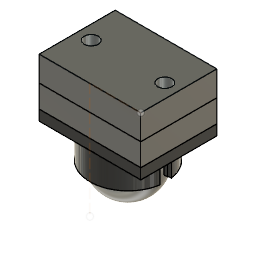
assembly (Autodesk Fusion 360 archive; units mm, degrees)
design "koło podporowe"
part number: 2025-11-20-20-36-54-064
part number: 2025-11-27-20-49-43-989
part number: 2025-11-27-20-56-08-265
Autodesk Fusion 360 part; units mm, degrees
note: some values were not read from the file. Set by a fixed rule: which face or edge a step refers to.
sketch "Szkic1" plane through (0, 0, 0) normal (0, 0, 1) x (1, 0, 0)
  line L0 (0, 0) -> (20.3, 0)
  line L1 (20.3, 0) -> (20.3, 15.2)
  line L2 (20.3, 15.2) -> (0, 15.2)
  line L3 (0, 15.2) -> (0, 0)
  dimension "d1" = 20.3
  dimension "d2" = 15.2
  constraint horizontal L0
  constraint vertical L1
  constraint horizontal L2
  constraint vertical L3
  constraint coincident L0.start L3.end
  measures "d1" distance of L0.start L0.end
  measures "d2" distance of L0.start L2.end
extrude "Wyciągnięcie proste1" add sketch "Szkic1" along normal blind 2.1 makes body 1
sketch "Szkic2" plane through (0, 0, 0) normal (0, 0, -1) x (1, 0, 0)
  line L0 (0, 0) -> (0, -15.2)
  line L1 (0, -15.2) -> (20.3, -15.2)
  line L2 (20.3, -15.2) -> (20.3, 0)
  line L3 (20.3, 0) -> (0, 0)
  circle A0 centre (2.8, -7.6) radius 1.15
  circle A1 centre (17.5, -7.6) radius 1.15
  dimension "d5" = 2.3
  dimension "d8" = 2.3
  measures "d5" diameter of A0
  measures "d8" diameter of A1
extrude "Wyciągnięcie proste2" cut sketch "Szkic2" against normal blind 4 contours A0 | A1 bodies 1
sketch "Szkic3" plane through (0, 0, 2.1) normal (0, 0, 1) x (-1, 0, 0)
  circle A0 centre (-2.8, -7.6) radius 1.15
  circle A1 centre (-17.5, -7.6) radius 1.15
  line L0 (0, -15.2) -> (0, 0)
  line L1 (0, 0) -> (-20.3, 0)
  line L2 (-20.3, 0) -> (-20.3, -15.2)
  line L3 (-20.3, -15.2) -> (0, -15.2)
  arc A2 (-17.6643, -8.7382) -> (-2.6357, -8.7382) centre (-10.15, -7.6) ccw
  arc A3 (-2.6357, -6.4618) -> (-17.6643, -6.4618) centre (-10.15, -7.6) ccw
  arc A4 (-3.9211, -6.6565) -> (-16.3789, -6.6565) centre (-10.15, -7.6) ccw
  arc A5 (-16.3789, -8.5435) -> (-3.9211, -8.5435) centre (-10.15, -7.6) ccw
  line L4 (-3.9211, -8.5435) -> (-3.294, -8.6385)
  line L5 (-3.9211, -6.6565) -> (-3.294, -6.5615)
  line L6 (-17.006, -6.5615) -> (-16.3789, -6.6565)
  line L7 (-17.006, -8.6385) -> (-16.3789, -8.5435)
  dimension "d13" = 15.2
  constraint coincident A1 A3.end
  constraint coincident A1 A2.start
  constraint coincident A0 A2.end
  constraint coincident A0 A3.start
  constraint concentric A2 A3
  constraint parallel L4 L6
  constraint parallel L5 L7
  constraint coincident A0 L4.end
  constraint coincident A0 L5.end
  constraint coincident A1 L7.start
  constraint coincident A1 L6.start
  measures "d13" diameter of A2
extrude "Wyciągnięcie proste3" add sketch "Szkic3" along normal blind 5.4 contours A0 A1 A3 A4 L5 L6 | A0 A1 A2 A5 L4 L7 bodies 1
sketch "Szkic4" plane through (0, 0, 0) normal (0, 0, -1) x (1, 0, 0)
  circle A0 centre (2.8, -7.6) radius 1.15
  circle A1 centre (17.5, -7.6) radius 1.15
  line L0 (0, 0) -> (0, -15.2)
  line L1 (0, -15.2) -> (20.3, -15.2)
  line L2 (20.3, -15.2) -> (20.3, 0)
  line L3 (20.3, 0) -> (0, 0)
  circle A2 centre (10.15, -7.6) radius 3.8
  dimension "d20" = 7.6
  measures "d20" diameter of A2
extrude "Wyciągnięcie proste4" cut sketch "Szkic4" against normal blind 4 contours A2 bodies 1
sphere "Prymityw sfery1" cut diameter 12.7 placed x (1, 0, 0) y (0, -1, 0) z (0, 0, -1) at (10.15, 7.6, 0) bodies 1
sphere "Prymityw sfery2" add diameter 12.7 placed x (1, 0, 0) y (0, -1, 0) z (0, 0, -1) at (10.15, 7.0726, 0) separate body makes body 2
move_body "Przesuń powierzchnię1" bodies 2 to x (1, 0, 0) y (0, 1, 0) z (0, 0, 1) at (0, 0, 7.15) on bodies 2
move_body "Przesuń powierzchnię2" bodies 2 to x (1, 0, 0) y (0, 1, 0) z (0, 0, 1) at (0, 0.5, 0) on bodies 2
sketch "Szkic7" plane through (0, 0, 0) normal (0, 1, 0) x (1, 0, 0)
sketch "Szkic8" plane through (0, 0, 0) normal (0, 0, 1) x (1, 0, 0)
  line L0 (0, 0) -> (20.3, 0)
  line L1 (20.3, 0) -> (20.3, 15.2)
  line L2 (20.3, 15.2) -> (0, 15.2)
  line L3 (0, 15.2) -> (0, 0)
  circle A0 centre (2.8, 7.6) radius 1.15
  arc A1 (3.8219, 8.1274) -> (3.8219, 7.0726) centre (2.8, 7.6) ccw
  circle A2 centre (17.5, 7.6) radius 1.15
  arc A3 (16.4781, 7.0726) -> (16.4781, 8.1274) centre (17.5, 7.6) ccw
  dimension "d27" = 20.3
  dimension "d28" = 15.2
  constraint horizontal L0
  constraint vertical L1
  constraint horizontal L2
  constraint vertical L3
  constraint coincident L0.start L3.end
  constraint tangent A0 A1
  constraint tangent A2 A3
  measures "d27" distance of L0.start L0.end
  measures "d28" distance of L0.start L2.end
ref_plane "Płaszczyzna konstrukcyjna1" through (10.15, 7.6, -1.5) normal (0, 0, -1) x (-1, 0, 0)
sketch "Szkic9" plane through (0, 0, -1.5) normal (0, 0, -1) x (-1, 0, 0)
  line L0 (0, 0) -> (-20.3, 0)
  line L1 (-20.3, 0) -> (-20.3, 15.2)
  line L2 (-20.3, 15.2) -> (0, 15.2)
  line L3 (0, 15.2) -> (0, 0)
  dimension "d32" = 20.3
  dimension "d33" = 15.2
  constraint horizontal L0
  constraint vertical L1
  constraint horizontal L2
  constraint vertical L3
  constraint coincident L0.start L3.end
  measures "d32" distance of L0.start L0.end
  measures "d33" distance of L0.start L2.end
extrude "Wyciągnięcie proste1'" add sketch "Szkic8" against normal blind 4.5 separate body makes body 3 in component "Component'"
ref_plane "Płaszczyzna konstrukcyjna2" through (10.15, 7.6, -4.5) normal (0, 0, -1) x (-1, 0, 0)
sketch "Szkic10" plane through (0, 0, -4.5) normal (0, 0, -1) x (-1, 0, 0)
  circle A0 centre (-2.8, 7.6) radius 1.4
  circle A1 centre (-17.5, 7.6) radius 1.4
  circle A2 centre (-17.5, 7.6) radius 1.15
  line L0 (-20.3, 0) -> (0, 0)
  line L1 (0, 0) -> (0, 15.2)
  line L2 (0, 15.2) -> (-20.3, 15.2)
  line L3 (-20.3, 15.2) -> (-20.3, 0)
  dimension "d39" = 2.8
  dimension "d40" = 2.8
  dimension "d41" = 20.3
  dimension "d42" = 15.2
  constraint concentric A1 A2
  constraint horizontal L0
  constraint vertical L1
  constraint horizontal L2
  constraint vertical L3
  measures "d39" diameter of A0
  measures "d40" diameter of A1
  measures "d41" distance of L0.start L0.end
  measures "d42" distance of L0.start L2.end
extrude "Wyciągnięcie proste1''" add sketch "Szkic10" along normal blind 5 separate body contours L0 L1 L2 L3 makes body 4 in component "do_druku"
move_body "Przesuń1" bodies 1 2 to x (-1, 0, 0) y (0, 1, 0) z (0, 0, -1) at (20.3, 0, 14.2)
move_body "Przesuń1'" bodies 4 to x (-1, 0, 0) y (0, 1, 0) z (0, 0, -1) at (20.3, 0, 14.2) in component "do_druku"
move_body "Przesuń1''" bodies 3 to x (-1, 0, 0) y (0, 1, 0) z (0, 0, -1) at (20.3, 0, 14.2) in component "Component'"
sketch "Szkic11" plane through (0, 0, 0) normal (0, 1, 0) x (1, 0, 0)
  line L0 (20.3, -23.7) -> (10.15, -23.7) construction
  line L1 (10.15, -23.7) -> (10.15, -0.7) construction
  dimension "d45" = 10.15
  dimension "d46" = 23
  constraint horizontal L0
  constraint vertical L1
  measures "d45" distance of L0.start L0.end
  measures "d46" distance of L0.end L1.end
sketch "Szkic12" plane through (0, 0, 23.7) normal (0, 0, 1) x (-1, 0, 0)
  circle A0 centre (-2.8, -7.6) radius 1.4
  circle A1 centre (-17.5, -7.6) radius 1.4
  line L0 (0, -15.2) -> (0, 0)
  line L1 (0, 0) -> (-20.3, 0)
  line L2 (-20.3, 0) -> (-20.3, -15.2)
  line L3 (-20.3, -15.2) -> (0, -15.2)
sketch "Szkic13" plane through (0, 0, 0) normal (0, 1, 0) x (1, 0, 0)
component "Component'" placed x (1, 0, 0) y (0, 1, 0) z (0, 0, 1) at (0, 0, 0)
component "do_druku" placed x (1, 0, 0) y (0, 1, 0) z (0, 0, 1) at (0, 0, 0)
named bodies: "kolo podporowe"

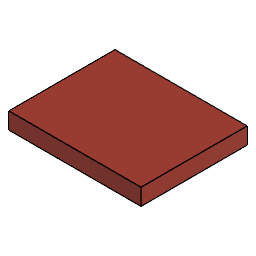
design "stepdown_5V"
part number: 2025-11-21-11-59-02-291
part number: 2025-11-29-20-27-12-206
Autodesk Fusion 360 part; units mm, degrees
sketch "Szkic1" plane through (0, 0, 0) normal (0, 0, 1) x (1, 0, 0)
  line L0 (0, 0) -> (12.7, 0)
  line L1 (12.7, 0) -> (12.7, 10.2)
  line L2 (12.7, 10.2) -> (0, 10.2)
  line L3 (0, 10.2) -> (0, 0)
  dimension "d1" = 12.7
  dimension "d2" = 10.2
  constraint horizontal L0
  constraint vertical L1
  constraint horizontal L2
  constraint vertical L3
  constraint coincident L0.start L3.end
  measures "d1" distance of L0.start L0.end
  measures "d2" distance of L0.start L2.end
extrude "Wyciągnięcie proste1" add sketch "Szkic1" along normal blind 1.6 makes body 1
copy_body "Bryła->Komponent1" bodies 1 removing the originals makes body 2 in component "Component"
component "Component" placed x (1, 0, 0) y (0, 1, 0) z (0, 0, 1) at (0, 0, 0)

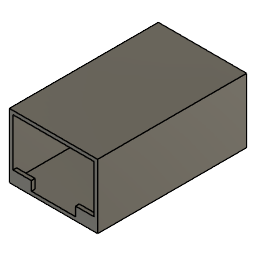
design "koszyk na koszyk"
part number: 2025-11-27-19-42-51-452
part number: 2025-11-29-21-01-25-605
Autodesk Fusion 360 part; units mm, degrees
sketch "Szkic1" plane through (0, 0, 0) normal (0, 0, 1) x (1, 0, 0)
  line L0 (0, 0) -> (48, 0)
  line L1 (48, 0) -> (48, 81)
  line L2 (48, 81) -> (0, 81)
  line L3 (0, 81) -> (0, 0)
  dimension "d1" = 48
  dimension "d2" = 81
  constraint horizontal L0
  constraint vertical L1
  constraint horizontal L2
  constraint vertical L3
  constraint coincident L0.start L3.end
  measures "d1" distance of L0.start L0.end
  measures "d2" distance of L0.start L2.end
extrude "Wyciągnięcie proste1" add sketch "Szkic1" along normal blind 2 makes body 1
ref_plane "Płaszczyzna konstrukcyjna1" through (0, 0, 2) normal (0, 0, 1) x (1, 0, 0)
sketch "Szkic2" plane through (0, 0, 2) normal (0, 0, 1) x (1, 0, 0)
  line L0 (0, 2) -> (2, 2) construction
  line L1 (0, 0) -> (48, 0)
  line L2 (48, 0) -> (48, 81)
  line L3 (48, 81) -> (0, 81)
  line L4 (0, 81) -> (0, 0)
  line L5 (2, 2) -> (12, 2)
  line L6 (12, 2) -> (12, 0)
  line L7 (12, 0) -> (2, 0)
  line L8 (2, 0) -> (2, 2)
  line L9 (46, 2) -> (36, 2)
  line L10 (36, 2) -> (36, 0)
  line L11 (36, 0) -> (46, 0)
  line L12 (46, 0) -> (46, 2)
  line L13 (0, 0) -> (2, 0)
  line L14 (2, 0) -> (2, 81)
  line L15 (2, 81) -> (0, 81)
  line L16 (0, 81) -> (0, 0)
  line L17 (48, 0) -> (46, 0)
  line L18 (46, 0) -> (46, 81)
  line L19 (46, 81) -> (48, 81)
  line L20 (48, 81) -> (48, 0)
  dimension "d8" = 44
  dimension "d10" = 48
  dimension "d11" = 81
  dimension "d12" = 10
  dimension "d13" = 2
  dimension "d16" = 10
  dimension "d19" = 81
  dimension "d22" = 81
  constraint horizontal L1
  constraint vertical L2
  constraint horizontal L3
  constraint vertical L4
  constraint coincident L1.start L4.end
  constraint horizontal L5
  constraint vertical L6
  constraint horizontal L7
  constraint vertical L8
  constraint horizontal L9
  constraint vertical L10
  constraint horizontal L11
  constraint vertical L12
  constraint horizontal L13
  constraint vertical L14
  constraint horizontal L15
  constraint vertical L16
  constraint horizontal L17
  constraint vertical L18
  constraint horizontal L19
  constraint vertical L20
  measures "d8" distance of L0.end L9.start
  measures "d10" distance of L1.start L1.end
  measures "d11" distance of L1.start L3.end
  measures "d12" distance of L0.end L5.end
  measures "d13" distance of L0.end L7.end
  measures "d16" distance of L9.start L9.end
  measures "d19" distance of L1.start L3.end
  measures "d22" distance of L1.end L2.end
extrude "Wyciągnięcie proste2" add sketch "Szkic2" along normal blind 5 contours L1 L5 L6 L7 L8 L14 bodies 1
extrude "Wyciągnięcie proste3" add sketch "Szkic2" along normal blind 5 contours L1 L9 L10 L11 L12 L18 bodies 1
extrude "Wyciągnięcie proste4" add sketch "Szkic2" along normal blind 31 contours L1 L3 L4 L8 L13 L14 L15 L16 bodies 1
extrude "Wyciągnięcie proste5" add sketch "Szkic2" along normal blind 31 contours L1 L2 L3 L12 L17 L18 L19 L20 bodies 1
ref_plane "Płaszczyzna konstrukcyjna2" through (0, 0, 33) normal (0, 0, 1) x (1, 0, 0)
sketch "Szkic3" plane through (0, 0, 33) normal (0, 0, 1) x (1, 0, 0)
  line L0 (0, 0) -> (48, 0)
  line L1 (48, 0) -> (48, 81)
  line L2 (48, 81) -> (0, 81)
  line L3 (0, 81) -> (0, 0)
  dimension "d26" = 48
  dimension "d27" = 81
  constraint horizontal L0
  constraint vertical L1
  constraint horizontal L2
  constraint vertical L3
  constraint coincident L0.start L3.end
  measures "d26" distance of L0.start L0.end
  measures "d27" distance of L0.start L2.end
extrude "Wyciągnięcie proste6" add sketch "Szkic3" along normal blind 2 bodies 1
copy_body "Bryła->Komponent1" bodies 1 removing the originals makes body 2 in component "Component"
component "Component" placed x (1, 0, 0) y (0, 1, 0) z (0, 0, 1) at (0, 0, 0)

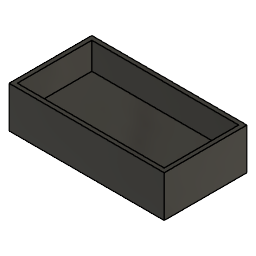
design "koszyk na baterie"
part number: 2025-11-20-20-18-58-786
part number: 2025-11-29-21-09-07-415
Autodesk Fusion 360 part; units mm, degrees
sketch "Szkic1" plane through (0, 0, 0) normal (0, 0, 1) x (1, 0, 0)
  line L0 (0, 0) -> (75, 0)
  line L1 (75, 0) -> (75, 40)
  line L2 (75, 40) -> (0, 40)
  line L3 (0, 40) -> (0, 0)
  dimension "d1" = 75
  dimension "d2" = 40
  constraint horizontal L0
  constraint vertical L1
  constraint horizontal L2
  constraint vertical L3
  constraint coincident L0.start L3.end
  measures "d1" distance of L0.start L0.end
  measures "d2" distance of L0.start L2.end
extrude "Wyciągnięcie proste1" add sketch "Szkic1" along normal blind 20 makes body 1
shell "Skorupa1" thickness 2 removed faces 1 at (25, 26.6667, 20) on bodies 1
extrude "Wyciągnięcie proste2" add 1 faces at (25.6667, 14, 2) along direction (0, 0, 1) blind 5 on bodies 1 bodies 1
copy_body "Bryła->Komponent1" bodies 1 removing the originals makes body 2 in component "koszyk"
component "koszyk" placed x (1, 0, 0) y (0, 1, 0) z (0, 0, 1) at (0, 0, 0)
named bodies: "koszyk"

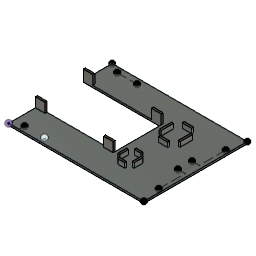
design "Podstawa"
part number: 2025-11-28-16-54-35-976
part number: 2025-11-29-20-28-41-836
Autodesk Fusion 360 part; units mm, degrees
other "Kontekst pochodny1"
sketch "Szkic1" plane through (0, 0, 0) normal (0, 0, 1) x (1, 0, 0)
  line L0 (0, 0) -> (141, 0)
  line L1 (141, 0) -> (141, 108)
  line L2 (141, 108) -> (0, 108)
  line L3 (0, 108) -> (0, 78)
  line L4 (0, 78) -> (81, 78)
  line L5 (81, 78) -> (81, 30)
  line L6 (81, 30) -> (0, 30)
  line L7 (0, 30) -> (0, 0)
  dimension "d1" = 141
  dimension "d2" = 108
  dimension "d3" = 141
  dimension "d4" = 30
  dimension "d5" = 81
  dimension "d6" = 48
  dimension "d7" = 81
  constraint coincident L0.start L7.end
  constraint horizontal L0
  constraint vertical L1
  constraint perpendicular L1 L2
  constraint perpendicular L2 L3
  constraint perpendicular L3 L4
  constraint vertical L5
  constraint perpendicular L5 L6
  measures "d1" distance of L0.start L0.end
  measures "d2" distance of L0.end L1.end
  measures "d3" distance of L1.end L2.end
  measures "d4" distance of L2.end L3.end
  measures "d5" distance of L3.end L4.end
  measures "d6" distance of L4.end L5.end
  measures "d7" distance of L5.end L6.end
extrude "Wyciągnięcie proste1" add sketch "Szkic1" against normal blind 2 makes body 1
sketch "Szkic2" plane through (0, 0, 0) normal (0, 0, 1) x (1, 0, 0)
  line L0 (0, 30) -> (10, 30)
  line L1 (10, 30) -> (10, 28)
  line L2 (10, 28) -> (0, 28)
  line L3 (0, 28) -> (0, 30)
  line L4 (0, 78) -> (10, 78)
  line L5 (10, 78) -> (10, 80)
  line L6 (10, 80) -> (0, 80)
  line L7 (0, 80) -> (0, 78)
  line L8 (81, 30) -> (71, 30)
  line L9 (71, 30) -> (71, 28)
  line L10 (71, 28) -> (81, 28)
  line L11 (81, 28) -> (81, 30)
  line L12 (81, 78) -> (71, 78)
  line L13 (71, 78) -> (71, 80)
  line L14 (71, 80) -> (81, 80)
  line L15 (81, 80) -> (81, 78)
  point P0 (81, 30)
  point P1 (81, 78)
  dimension "d10" = 10
  dimension "d11" = 2
  dimension "d12" = 10
  dimension "d13" = 2
  dimension "d14" = 10
  dimension "d15" = 2
  dimension "d16" = 10
  dimension "d17" = 2
  constraint horizontal L0
  constraint vertical L1
  constraint horizontal L2
  constraint vertical L3
  constraint horizontal L4
  constraint vertical L5
  constraint horizontal L6
  constraint vertical L7
  constraint horizontal L8
  constraint vertical L9
  constraint horizontal L10
  constraint vertical L11
  constraint coincident P0 L8.start
  constraint horizontal L12
  constraint vertical L13
  constraint horizontal L14
  constraint vertical L15
  constraint coincident P1 L12.start
  measures "d10" distance of L0.start L0.end
  measures "d11" distance of L0.start L2.end
  measures "d12" distance of L4.start L4.end
  measures "d13" distance of L4.start L6.end
  measures "d14" distance of P0 L8.end
  measures "d15" distance of P0 L10.end
  measures "d16" distance of P1 L12.end
  measures "d17" distance of P1 L14.end
extrude "Wyciągnięcie proste2" add sketch "Szkic2" along normal blind 10 contours L0 L1 L2 L3 bodies 1
extrude "Wyciągnięcie proste3" add sketch "Szkic2" along normal blind 10 contours L4 L5 L6 L7 | L8 L9 L10 L11 | L12 L13 L14 L15 bodies 1
sketch "Szkic3" plane through (0, 0, 0) normal (0, 0, 1) x (1, 0, 0)
  line L0 (81, 78) -> (81, 30)
  line L1 (81, 54) -> (89, 54) construction
  line L2 (89, 54) -> (89, 108) construction
  line L3 (89, 108) -> (89, 81) construction
  line L4 (89, 81) -> (91, 81)
  line L5 (91, 81) -> (91, 68)
  line L6 (91, 68) -> (89, 68)
  line L7 (89, 68) -> (89, 81)
  line L8 (91, 81) -> (95, 81) construction
  line L9 (95, 81) -> (95, 86) construction
  line L10 (95, 86) -> (105, 86)
  line L11 (105, 86) -> (105, 88)
  line L12 (105, 88) -> (95, 88)
  line L13 (95, 88) -> (95, 86)
  line L14 (91, 68) -> (95, 68) construction
  line L15 (95, 68) -> (95, 63) construction
  line L16 (95, 63) -> (105, 63)
  line L17 (105, 63) -> (105, 61)
  line L18 (105, 61) -> (95, 61)
  line L19 (95, 61) -> (95, 63)
  line L20 (105, 63) -> (109, 63) construction
  line L21 (109, 63) -> (109, 68) construction
  line L22 (109, 68) -> (111, 68)
  line L23 (111, 68) -> (111, 81)
  line L24 (111, 81) -> (109, 81)
  line L25 (109, 81) -> (109, 68)
  line L26 (95, 61) -> (95, 39) construction
  line L27 (95, 39) -> (94, 39) construction
  line L28 (94, 39) -> (101, 39)
  line L29 (101, 39) -> (101, 37)
  line L30 (101, 37) -> (94, 37)
  line L31 (94, 37) -> (94, 39)
  line L32 (94, 37) -> (94, 34) construction
  line L33 (94, 34) -> (91, 34) construction
  line L34 (91, 34) -> (89, 34)
  line L35 (89, 34) -> (89, 25)
  line L36 (89, 25) -> (91, 25)
  line L37 (91, 25) -> (91, 34)
  line L38 (91, 25) -> (94, 25) construction
  line L39 (94, 25) -> (94, 22) construction
  line L40 (94, 22) -> (101, 22)
  line L41 (101, 22) -> (101, 20)
  line L42 (101, 20) -> (94, 20)
  line L43 (94, 20) -> (94, 22)
  line L44 (101, 22) -> (104, 22) construction
  line L45 (104, 22) -> (104, 25) construction
  line L46 (104, 25) -> (106, 25)
  line L47 (106, 25) -> (106, 34)
  line L48 (106, 34) -> (104, 34)
  line L49 (104, 34) -> (104, 25)
  dimension "d22" = 8
  dimension "d23" = 27
  dimension "d24" = 13
  dimension "d25" = 4
  dimension "d26" = 5
  dimension "d27" = 10
  dimension "d28" = 2
  dimension "d29" = 4
  dimension "d30" = 5
  dimension "d31" = 10
  dimension "d32" = 2
  dimension "d33" = 4
  dimension "d34" = 5
  dimension "d35" = 2
  dimension "d36" = 13
  dimension "d39" = 22
  dimension "d40" = 1
  dimension "d41" = 7
  dimension "d42" = 2
  dimension "d43" = 3
  dimension "d44" = 3
  dimension "d45" = 2
  dimension "d46" = 9
  dimension "d47" = 3
  dimension "d48" = 3
  dimension "d49" = 7
  dimension "d50" = 2
  dimension "d51" = 3
  dimension "d52" = 3
  dimension "d53" = 2
  dimension "d54" = 9
  constraint midpoint L0 L1.start
  constraint perpendicular L0 L1
  constraint perpendicular L1 L2
  constraint parallel L2 L3
  constraint horizontal L4
  constraint vertical L5
  constraint horizontal L6
  constraint vertical L7
  constraint perpendicular L5 L8
  constraint perpendicular L8 L9
  constraint horizontal L10
  constraint vertical L11
  constraint horizontal L12
  constraint vertical L13
  constraint horizontal L14
  constraint perpendicular L14 L15
  constraint horizontal L16
  constraint vertical L17
  constraint horizontal L18
  constraint vertical L19
  constraint perpendicular L17 L20
  constraint perpendicular L20 L21
  constraint horizontal L22
  constraint vertical L23
  constraint horizontal L24
  constraint vertical L25
  constraint perpendicular L18 L26
  constraint perpendicular L0 L27
  constraint horizontal L28
  constraint vertical L29
  constraint horizontal L30
  constraint vertical L31
  constraint perpendicular L30 L32
  constraint horizontal L33
  constraint horizontal L34
  constraint vertical L35
  constraint horizontal L36
  constraint vertical L37
  constraint perpendicular L37 L38
  constraint perpendicular L38 L39
  constraint horizontal L40
  constraint vertical L41
  constraint horizontal L42
  constraint vertical L43
  constraint perpendicular L41 L44
  constraint perpendicular L44 L45
  constraint horizontal L46
  constraint vertical L47
  constraint horizontal L48
  constraint vertical L49
  measures "d22" distance of L1.start L1.end
  measures "d23" distance of L2.end L3.end
  measures "d24" distance of L3.end L6.end
  measures "d25" distance of L4.end L8.end
  measures "d26" distance of L8.end L9.end
  measures "d27" distance of L9.end L10.end
  measures "d28" distance of L9.end L12.end
  measures "d29" distance of L5.end L14.end
  measures "d30" distance of L14.end L15.end
  measures "d31" distance of L15.end L16.end
  measures "d32" distance of L15.end L18.end
  measures "d33" distance of L16.end L20.end
  measures "d34" distance of L20.end L21.end
  measures "d35" distance of L21.end L22.end
  measures "d36" distance of L21.end L24.end
  measures "d39" distance of L18.end L26.end
  measures "d40" distance of L26.end L27.end
  measures "d41" distance of L27.end L28.end
  measures "d42" distance of L27.end L30.end
  measures "d43" distance of L30.end L32.end
  measures "d44" distance of L32.end L33.end
  measures "d45" distance of L33.end L34.end
  measures "d46" distance of L33.end L36.end
  measures "d47" distance of L36.end L38.end
  measures "d48" distance of L38.end L39.end
  measures "d49" distance of L39.end L40.end
  measures "d50" distance of L39.end L42.end
  measures "d51" distance of L40.end L44.end
  measures "d52" distance of L44.end L45.end
  measures "d53" distance of L45.end L46.end
  measures "d54" distance of L45.end L48.end
extrude "Wyciągnięcie proste4" add sketch "Szkic3" along normal blind 5 contours L4 L5 L6 L7 | L10 L11 L12 L13 | L16 L17 L18 L19 | L22 L23 L24 L25 bodies 1
extrude "Wyciągnięcie proste5" add sketch "Szkic3" along normal blind 5 contours L28 L29 L30 L31 | L34 L35 L36 L37 | L40 L41 L42 L43 | L46 L47 L48 L49 bodies 1
copy_body "Bryła->Komponent1" bodies 1 removing the originals makes body 2 in component "Component"
sketch "Szkic5" plane through (0, 0, 0) normal (0, 0, 1) x (-1, 0, 0)
  line L0 (-94, -20) -> (-94, -22)
  line L1 (-94, -22) -> (-101, -22)
  line L2 (-101, -22) -> (-101, -20)
  line L3 (-101, -20) -> (-94, -20)
  line L4 (-104, -34) -> (-106, -34)
  line L5 (-106, -34) -> (-106, -25)
  line L6 (-106, -25) -> (-104, -25)
  line L7 (-104, -25) -> (-104, -34)
  line L8 (-91, -25) -> (-89, -25)
  line L9 (-89, -25) -> (-89, -34)
  line L10 (-89, -34) -> (-91, -34)
  line L11 (-91, -34) -> (-91, -25)
  line L12 (-94, -37) -> (-94, -39)
  line L13 (-94, -39) -> (-101, -39)
  line L14 (-101, -39) -> (-101, -37)
  line L15 (-101, -37) -> (-94, -37)
  line L16 (-95, -61) -> (-95, -63)
  line L17 (-95, -63) -> (-105, -63)
  line L18 (-105, -63) -> (-105, -61)
  line L19 (-105, -61) -> (-95, -61)
  line L20 (-89, -68) -> (-89, -81)
  line L21 (-89, -81) -> (-91, -81)
  line L22 (-91, -81) -> (-91, -68)
  line L23 (-91, -68) -> (-89, -68)
  line L24 (-109, -81) -> (-111, -81)
  line L25 (-111, -81) -> (-111, -68)
  line L26 (-111, -68) -> (-109, -68)
  line L27 (-109, -68) -> (-109, -81)
  line L28 (-95, -88) -> (-105, -88)
  line L29 (-105, -88) -> (-105, -86)
  line L30 (-105, -86) -> (-95, -86)
  line L31 (-95, -86) -> (-95, -88)
  line L32 (-71, -78) -> (-71, -80)
  line L33 (-71, -80) -> (-81, -80)
  line L34 (-81, -80) -> (-81, -78)
  line L35 (-81, -78) -> (-81, -30)
  line L36 (-81, -30) -> (-81, -28)
  line L37 (-81, -28) -> (-71, -28)
  line L38 (-71, -28) -> (-71, -30)
  line L39 (-71, -30) -> (-10, -30)
  line L40 (-10, -30) -> (-10, -28)
  line L41 (-10, -28) -> (0, -28)
  line L42 (0, -28) -> (0, 0)
  line L43 (0, 0) -> (-141, 0)
  line L44 (-141, 0) -> (-141, -108)
  line L45 (-141, -108) -> (0, -108)
  line L46 (0, -108) -> (0, -80)
  line L47 (0, -80) -> (-10, -80)
  line L48 (-10, -80) -> (-10, -78)
  line L49 (-10, -78) -> (-71, -78)
  line L50 (-141, 0) -> (-141, -19.075) construction
  line L51 (-141, -19.075) -> (-137.5, -19.075) construction
  circle A0 centre (-137.5, -19.075) radius 1.15
  line L52 (-141, -108) -> (-141, -88.925) construction
  line L53 (-141, -88.925) -> (-137.5, -88.925) construction
  circle A1 centre (-137.5, -88.925) radius 1.15
  line L54 (0, 0) -> (-10.9, 0) construction
  line L55 (-10.9, 0) -> (-10.9, -5.75) construction
  circle A2 centre (-10.9, -5.75) radius 1.15
  circle A3 centre (-31.7, -5.75) radius 1.15
  line L56 (0, -108) -> (-10.9, -108) construction
  line L57 (-10.9, -108) -> (-10.9, -102.25) construction
  circle A4 centre (-10.9, -102.25) radius 1.15
  line L58 (-10.9, -102.25) -> (-31.7, -102.25) construction
  circle A5 centre (-31.7, -102.25) radius 1.15
  line L59 (-137.5, -19.075) -> (-137.5, -46.65) construction
  line L60 (-137.5, -46.65) -> (-129.9, -46.65) construction
  line L61 (-137.5, -88.925) -> (-137.5, -61.35) construction
  line L62 (-137.5, -61.35) -> (-129.9, -61.35) construction
  circle A6 centre (-129.9, -61.35) radius 1.15
  circle A7 centre (-129.9, -46.65) radius 1.15
  dimension "d57" = 19.075
  dimension "d58" = 3.5
  dimension "d59" = 2.3
  dimension "d60" = 19.075
  dimension "d61" = 3.5
  dimension "d62" = 2.3
  dimension "d65" = 10.9
  dimension "d66" = 5.75
  dimension "d67" = 2.3
  dimension "d68" = 20.8
  dimension "d69" = 2.3
  dimension "d70" = 10.9
  dimension "d71" = 5.75
  dimension "d72" = 2.3
  dimension "d73" = 20.8
  dimension "d74" = 2.3
  dimension "d77" = 27.575
  dimension "d78" = 7.6
  dimension "d79" = 27.575
  dimension "d80" = 7.6
  dimension "d81" = 2.3
  dimension "d82" = 2.3
  constraint coincident L43.end L44.start
  constraint perpendicular L43 L50
  constraint perpendicular L50 L51
  constraint coincident L51.end A0.centre
  constraint coincident L44.end L45.start
  constraint perpendicular L45 L52
  constraint perpendicular L44 L53
  constraint coincident L53.end A1.centre
  constraint coincident L42.end L43.start
  constraint perpendicular L42 L54
  constraint perpendicular L54 L55
  constraint coincident L55.end A2.centre
  constraint coincident L45.end L46.start
  constraint perpendicular L46 L56
  constraint perpendicular L56 L57
  constraint coincident L57.end A4.centre
  constraint perpendicular L57 L58
  constraint coincident L58.end A5.centre
  constraint perpendicular L51 L59
  constraint perpendicular L59 L60
  constraint perpendicular L53 L61
  constraint perpendicular L61 L62
  constraint coincident L62.end A6.centre
  constraint coincident L60.end A7.centre
  measures "d57" distance of L43.end L50.end
  measures "d58" distance of L50.end L51.end
  measures "d59" diameter of A0
  measures "d60" distance of L44.end L52.end
  measures "d61" distance of L52.end L53.end
  measures "d62" diameter of A1
  measures "d65" distance of L42.end L54.end
  measures "d66" distance of L54.end L55.end
  measures "d67" diameter of A2
  measures "d68" distance of L55.end A3.centre
  measures "d69" diameter of A3
  measures "d70" distance of L45.end L56.end
  measures "d71" distance of L56.end L57.end
  measures "d72" diameter of A4
  measures "d73" distance of L57.end L58.end
  measures "d74" diameter of A5
  measures "d77" distance of L51.end L59.end
  measures "d78" distance of L59.end L60.end
  measures "d79" distance of L53.end L61.end
  measures "d80" distance of L61.end L62.end
  measures "d81" diameter of A6
  measures "d82" diameter of A7
extrude "Wyciągnięcie proste1'" cut sketch "Szkic5" against normal blind 2 contours A0 | A1 bodies 2 in component "Component"
extrude "Wyciągnięcie proste2'" cut sketch "Szkic5" against normal blind 2 contours A2 | A3 | A4 | A5 bodies 2 in component "Component"
extrude "Wyciągnięcie proste3'" cut sketch "Szkic5" against normal blind 2 contours A6 | A7 bodies 2 in component "Component"
component "Component" placed x (1, 0, 0) y (0, 1, 0) z (0, 0, 1) at (0, 0, 0)

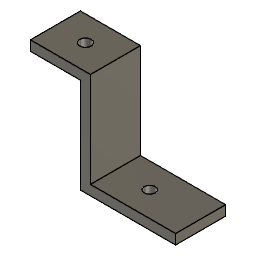
design "mocowanie czujnik"
part number: 2025-11-28-17-20-17-522
part number: 2025-11-28-17-33-48-723
Autodesk Fusion 360 part; units mm, degrees
other "Kontekst pochodny1"
sketch "Szkic1" plane through (0, 0, 0) normal (0, 0, 1) x (1, 0, 0)
  line L0 (0, 0) -> (12, 0)
  line L1 (12, 0) -> (12, -19)
  line L2 (12, -19) -> (29, -19)
  line L3 (29, -19) -> (29, -21)
  line L4 (29, -21) -> (10, -21)
  line L5 (10, -21) -> (10, -2)
  line L6 (10, -2) -> (0, -2)
  line L7 (0, -2) -> (0, 0)
  dimension "d1" = 12
  dimension "d2" = 19
  dimension "d3" = 17
  dimension "d4" = 2
  dimension "d5" = 19
  dimension "d6" = 19
  dimension "d7" = 10
  dimension "d8" = 2
  constraint coincident L0.start L7.end
  constraint horizontal L0
  constraint perpendicular L0 L1
  constraint perpendicular L1 L2
  constraint perpendicular L2 L3
  constraint perpendicular L3 L4
  constraint vertical L5
  constraint perpendicular L5 L6
  measures "d1" distance of L0.start L0.end
  measures "d2" distance of L0.end L1.end
  measures "d3" distance of L1.end L2.end
  measures "d4" distance of L2.end L3.end
  measures "d5" distance of L3.end L4.end
  measures "d6" distance of L4.end L5.end L2.end
  measures "d7" distance of L5.end L6.end L2.end
  measures "d8" distance of L6.end L0.start
extrude "Wyciągnięcie proste1" add sketch "Szkic1" along normal blind 10 makes body 1
copy_body "Bryła->Komponent1" bodies 1 removing the originals makes body 2 in component "Component"
move_body "Przesuń1" bodies 2 to x (1, 0, 0) y (0, 0, 1) z (0, -1, 0) at (0, -21, 21) in component "Component"
sketch "Szkic2" plane through (0, 0, 0) normal (0, 0, 1) x (1, 0, 0)
  line L0 (29, -21) -> (29, -26) construction
  line L1 (29, -26) -> (18.84, -26) construction
  circle A0 centre (18.84, -26) radius 1.092
  dimension "d11" = 5
  dimension "d12" = 10.16
  dimension "d13" = 2.184
  constraint vertical L0
  constraint perpendicular L0 L1
  constraint coincident L1.end A0.centre
  measures "d11" distance of L0.start L0.end
  measures "d12" distance of L0.end L1.end
  measures "d13" diameter of A0
extrude "Wyciągnięcie proste1'" cut sketch "Szkic2" along normal blind 2 bodies 2 in component "Component"
sketch "Szkic3" plane through (0, 0, 21) normal (0, 0, 1) x (-1, 0, 0)
  line L0 (-12, 21) -> (0, 21)
  line L1 (0, 21) -> (0, 31)
  line L2 (0, 31) -> (-12, 31)
  line L3 (-12, 31) -> (-12, 21)
  line L4 (-12, 31) -> (0, 21) construction
  line L5 (-12, 21) -> (0, 31) construction
  circle A0 centre (-6, 26) radius 1.15
  dimension "d16" = 2.3
  constraint coincident L2.end L3.start
  constraint coincident L0.end L1.start
  constraint coincident L0.start L3.end
  constraint coincident L1.end L2.start
  constraint midpoint L5 A0.centre
  measures "d16" diameter of A0
extrude "Wyciągnięcie proste2" cut sketch "Szkic3" against normal blind 2 contours A0 bodies 2 in component "Component"
component "Component" placed x (1, 0, 0) y (0, 1, 0) z (0, 0, 1) at (0, 0, 0)

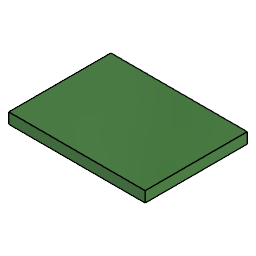
design "TB6612FNG"
part number: 2025-11-21-11-44-20-767
part number: 2025-11-29-20-31-23-735
Autodesk Fusion 360 part; units mm, degrees
sketch "Szkic1" plane through (0, 0, 0) normal (0, 0, 1) x (1, 0, 0)
  line L0 (0, 0) -> (20.3, 0)
  line L1 (20.3, 0) -> (20.3, 15.2)
  line L2 (20.3, 15.2) -> (0, 15.2)
  line L3 (0, 15.2) -> (0, 0)
  dimension "d1" = 20.3
  dimension "d2" = 15.2
  constraint horizontal L0
  constraint vertical L1
  constraint horizontal L2
  constraint vertical L3
  constraint coincident L0.start L3.end
  measures "d1" distance of L0.start L0.end
  measures "d2" distance of L0.start L2.end
extrude "Wyciągnięcie proste1" add sketch "Szkic1" along normal blind 1.6 makes body 1
copy_body "Bryła->Komponent1" bodies 1 removing the originals makes body 2 in component "Component"
component "Component" placed x (1, 0, 0) y (0, 1, 0) z (0, 0, 1) at (0, 0, 0)
